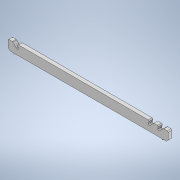
# Autodesk Inventor part: trunk 2
Saved by Autodesk Inventor 2020.1 (Build 241239000, 239)
## iProperties
Created: 2022-03-19
Part Number: trunk 2
Material: Типовые
Document SubType Name: Modeling
Designer: User
Density: 1 g/cm^3
Appearance: По умолчанию
Author: User
Autodesk Inventor part; units mm, degrees
ref_plane "YZ Plane" through (0, 0, 0) normal (1, 0, 0) x (0, 1, 0)
ref_plane "XZ Plane" through (0, 0, 0) normal (0, 1, 0) x (-1, 0, 0)
ref_plane "XY Plane" through (0, 0, 0) normal (0, 0, 1) x (1, 0, 0)
sketch "Эскиз1" plane through (0, 0, 0) normal (0, 0, 1) x (1, 0, 0)
  line L0 (0, 0) -> (-170, 0)
  line L1 (-170, 0) -> (-170, 10)
  line L2 (-170, 10) -> (0, 10)
  line L3 (0, 10) -> (0, 0)
  line L4 (-156.1916, 10) -> (-150.6349, 10) construction
  line L5 (-165, 10) -> (-158.1699, 3.1699)
  line L6 (-10, 10) -> (-34.5353, 10)
  line L7 (-30, 10) -> (-25, 10)
  line L8 (-23.8869, 10) -> (-18.8869, 10)
  line L9 (-15, 10) -> (-20, 10)
  line L10 (-170, 0) -> (-169, -1)
  line L11 (-170, 0) -> (-168.5858, 0) construction
  line L12 (-169, -1) -> (-169, 0)
  line L13 (-163.7026, 0) -> (-163.7026, -1)
  line L14 (-163.7026, -1) -> (-162.7026, 0)
  line L15 (0, 0) -> (-1, -1)
  line L16 (0, 0) -> (1.4142, 0) construction
  line L17 (-1, -1) -> (-1, 0)
  line L18 (-6, 0) -> (-6, -1)
  line L19 (-6, -1) -> (-7, 0)
  line L20 (-87, 0) -> (-87, -1)
  line L21 (-87, -1) -> (-88, 0)
  line L22 (-83, 0) -> (-83, -1)
  line L23 (-83, -1) -> (-82, 0)
  line L24 (-158.1699, 3.1699) -> (-160, 10)
  line L25 (-5, 10) -> (-11.8301, 3.1699)
  line L26 (-11.8301, 3.1699) -> (-10, 10)
  line L27 (-15, 10) -> (-21.8301, 3.1699)
  line L28 (-21.8301, 3.1699) -> (-20, 10)
  line L29 (-167.7026, 0) -> (-170, 2.2974)
  line L30 (-2, 0) -> (0, 2)
  point P0 (-170, 5)
  point P1 (-85, 0)
  point P2 (-161.5849, 6.5849)
  point P3 (-5, 10)
  point P4 (-15, 10)
  point P5 (-20, 10)
  dimension "d1" = 10
  dimension "d3" = 45
  dimension "d4" = 5
  dimension "d21" = 45
  dimension "d22" = 45
  dimension "d23" = 1
  dimension "d25" = 1
  dimension "d26" = 135
  dimension "d27" = 1
  dimension "d29" = 1
  dimension "d30" = 45
  dimension "d31" = 2
  dimension "d32" = 45
  dimension "d33" = 1
  dimension "d34" = 1
  dimension "d35" = 2
  dimension "d36" = 45
  dimension "d37" = 75
  dimension "d38" = 5
  dimension "d43" = 150
  dimension "d44" = 5
  dimension "d51" = 45
  dimension "d52" = 75
  dimension "d53" = 5
  dimension "d54" = 5
  dimension "d59" = 45
  dimension "d60" = 75
  dimension "d67" = 5
  dimension "d69" = 45
  dimension "d70" = 4
  dimension "d71" = 45
  dimension "d72" = 2
  dimension "d73" = 4
  constraints: 60 end point, 8 horizontal, 7 vertical, 6 point on line, 2 coincident, 2 equal length, 2 midpoint, 1 parallel, 16 other
  measures "d1" distance of L2.end L3.end
  measures "d3" angle of L5 L2
  measures "d4" distance of L5.start L1.end
  measures "d21" angle of L10 L11
  measures "d22" angle of L14 L13
  measures "d23" distance of L10.end L12.end
  measures "d25" distance of L13.start L13.end
  measures "d26" angle of L15 L16
  measures "d27" distance of L15.end L17.end
  measures "d29" distance of L18.start L18.end
  measures "d30" angle to the sketch x axis of L19
  measures "d31" distance of point (-85, 0) L20.start
  measures "d32" angle to the sketch x axis of L21
  measures "d33" distance of L20.start L20.end
  measures "d34" distance of L22.start L22.end
  measures "d35" distance of point (-85, 0) L22.start
  measures "d36" angle to the sketch x axis of L23
  measures "d37" angle of L2 L24
  measures "d38" distance of L24.end L5.start
  measures "d43" distance of L6.start L24.end
  measures "d44" distance of L6.start L25.start
  measures "d51" angle of L2 L25
  measures "d52" angle of L2 L26
  measures "d53" distance of L27.start L6.start
  measures "d54" distance of L28.end L27.start
  measures "d59" angle of L2 L27
  measures "d60" angle of L2 L28
  measures "d67" distance of L2.end L25.start
  measures "d69" angle to the sketch x axis of L29
  measures "d70" distance of L13.start L29.start
  measures "d71" angle to the sketch x axis of L30
  measures "d73" distance of L30.start L18.start
extrude "Выдавливание1" add sketch "Эскиз1" along normal blind 4 contours L30 L0 L29 L1 L2 L5 L24 L28 L27 L26 L25 L3 | L18 L19 L0 | L14 L13 L0
fillet "Сопряжение2" radius 1 2 edges at (0, 10, 2) (-170, 10, 2)
fillet "Сопряжение3" radius 1 8 edges at (-21.8301, 3.1699, 2) (-11.8301, 3.1699, 2) (-10, 10, 2) (-5, 10, 2) (-20, 10, 2) (-158.1699, 3.1699, 2) (-165, 10, 2) (-160, 10, 2)
